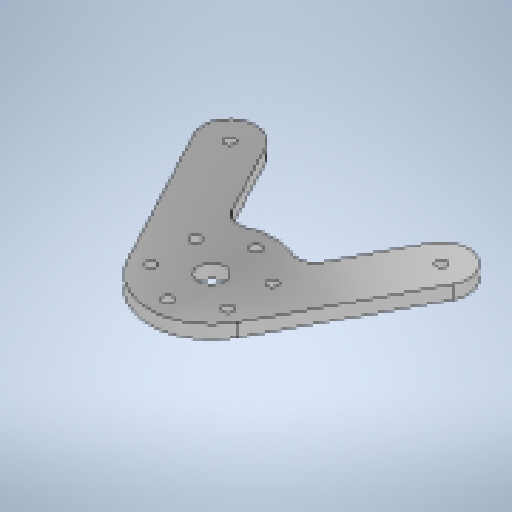
# Autodesk Inventor part: Upright - Bottom
Saved by Autodesk Inventor 2023.4 (Build 274418000, 418)
## iProperties
Created: 2024-09-12
Part Number: Upright - Bottom
Material: Aluminum 6061
Document SubType Name: Modeling
Designer: Nathan Cai
Mass: 41.5661 g
Surface Area: 85.6405 cm^2
Volume: 15.3949 cm^3
Density: 2.7 g/cm^3
Appearance: Aluminum - Flat
Author: Nathan Cai
Autodesk Inventor part; units mm, degrees
ref_plane "YZ Plane" through (0, 0, 0) normal (1, 0, 0) x (0, 1, 0)
ref_plane "XZ Plane" through (0, 0, 0) normal (0, 1, 0) x (-1, 0, 0)
ref_plane "XY Plane" through (0, 0, 0) normal (0, 0, 1) x (1, 0, 0)
sketch "Sketch1" plane through (0, 0, 0) normal (0, 1, 0) x (-1, 0, 0)
  circle A0 centre (0, 0) radius 38.1 construction
  line L0 (0, 0) -> (38.1, 0) construction
  line L1 (0, 0) -> (-38.1, 0) construction
  circle A1 centre (38.1, 0) radius 1.905
  circle A2 centre (-38.1, 0) radius 1.905
  circle A3 centre (38.1, 0) radius 9.525
  circle A4 centre (-38.1, 0) radius 9.525
  line L2 (0, 0) -> (0, 44.45) construction
  circle A5 centre (0, 44.45) radius 76.2 construction
  circle A6 centre (0, 44.45) radius 19.05 construction
  circle A7 centre (0, 0) radius 25.4 construction
  circle A8 centre (0, 44.45) radius 4.7625
  circle A9 centre (0, 44.45) radius 22.225
  line L3 (19.6103, 54.9088) -> (46.5044, 4.4824)
  line L4 (-19.6103, 54.9088) -> (-46.5044, 4.4824)
  line L5 (13.153, 26.535) -> (29.6956, -4.4824)
  line L6 (-13.153, 26.535) -> (-29.6956, -4.4824)
  circle A10 centre (0, 44.45) radius 15.875 construction
  circle A11 centre (0, 60.325) radius 1.905
  circle A12 centre (-13.7482, 52.3875) radius 1.905
  circle A13 centre (-13.7482, 36.5125) radius 1.905
  circle A14 centre (0, 28.575) radius 1.905
  circle A15 centre (13.7482, 36.5125) radius 1.905
  circle A16 centre (13.7482, 52.3875) radius 1.905
  point P0 (-29.6956, -4.4824)
  point P1 (29.6956, -4.4824)
  dimension "d3" = 19.05
  dimension "d14" = 31.75
  dimension "d0" = 76.2
  dimension "d1" = 3.81
  dimension "d2" = 3.81
  dimension "d4" = 19.05
  dimension "d5" = 152.4
  dimension "d6" = 38.1
  dimension "d7" = 50.8
  dimension "d8" = 9.525
  dimension "d9" = 44.45
  dimension "d10" = 19.05
  dimension "d15" = 3.81
  dimension "d18" = 360
  constraints: 15 centre point, 14 end point, 10 coincident, 4 point on circle, 4 symmetric about line, 2 point on line, 2 tangent, 1 horizontal, 1 parallel, 1 vertical, 1 vertical alignment, 19 other
  measures "d0" diameter of A0
  measures "d1" diameter of A1
  measures "d2" diameter of A2
  measures "d4" diameter of A4
  measures "d5" diameter of A5
  measures "d6" diameter of A6
  measures "d7" diameter of A7
  measures "d8" diameter of A8
  measures "d9" diameter of A9
  measures "d10" distance between parallel lines of L3 L5
  measures "d15" diameter of A11
extrude "Extrusion1" add sketch "Sketch1" along normal blind 4.7625
fillet "Fillet1" radius 6.35 2 edges at (-13.153, 2.3813, 26.535) (13.153, 2.3813, 26.535)
equation "\"d2\" = d1"
equation "\"d4\" = d3"
body "Solid1"
